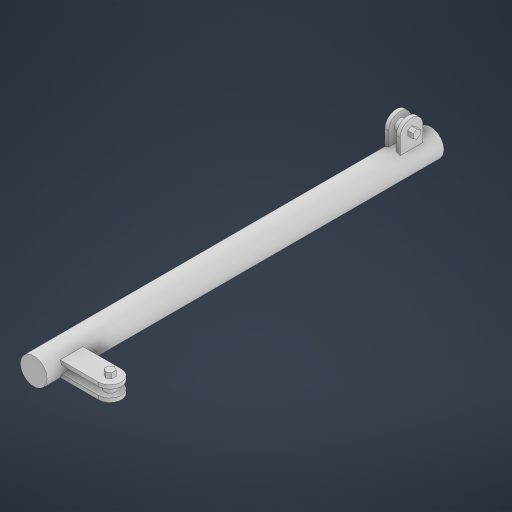
# Autodesk Inventor part: driveshaft_m_mount
Saved by Autodesk Inventor 2023 (Build 270158000, 158)
## iProperties
Created: 2023-09-20
Part Number: driveshaft_m_mount
Material: Generic
Document SubType Name: Modeling
Designer: Peter
Density: 1 g/cm^3
Appearance: Default
Author: Peter
Autodesk Inventor part; units mm, degrees
ref_plane "YZ Plane" through (0, 0, 0) normal (1, 0, 0) x (0, 1, 0)
ref_plane "XZ Plane" through (0, 0, 0) normal (0, 1, 0) x (-1, 0, 0)
ref_plane "XY Plane" through (0, 0, 0) normal (0, 0, 1) x (1, 0, 0)
sketch "Sketch1" plane through (0, 0, 0) normal (0, 0, 1) x (1, 0, 0)
  circle A0 centre (0, 0) radius 44.45
  dimension "d0" = 88.9
  constraints: 1 centre point, 1 coincident
  measures "d0" diameter of A0
extrude "Extrusion1" add sketch "Sketch1" along normal blind 1320.8
sketch "Sketch2" plane through (0, 0, 0) normal (0, 1, 0) x (-1, 0, 0)
  line L0 (12.7, 50.8) -> (25.4, 50.8)
  line L1 (25.4, 50.8) -> (25.4, 127)
  line L2 (25.4, 127) -> (12.7, 127)
  line L3 (12.7, 127) -> (12.7, 50.8)
  line L4 (0, -25.4) -> (0, 152.4) construction
  line L5 (-12.7, 50.8) -> (-25.4, 50.8)
  line L6 (-25.4, 50.8) -> (-25.4, 127)
  line L7 (-25.4, 127) -> (-12.7, 127)
  line L8 (-12.7, 127) -> (-12.7, 50.8)
  point P0 (0, 0)
  dimension "d3" = 76.2
  dimension "d4" = 12.7
  dimension "d5" = 12.7
  dimension "d6" = 50.8
  constraints: 16 end point, 4 symmetric about line, 2 parallel, 1 horizontal, 1 perpendicular
  measures "d3" distance of L0.end L1.end
  measures "d4" distance of L1.end L2.end
  measures "d5" distance between parallel lines of L4 L3
  measures "d6" distance from line of point (0, 0) L0
extrude "Extrusion2" add sketch "Sketch2" along normal blind 127
sketch "Sketch3" plane through (0, 0, 0) normal (1, 0, 0) x (0, 1, 0)
  line L0 (12.7, 1270) -> (25.4, 1270)
  line L1 (25.4, 1270) -> (25.4, 1193.8)
  line L2 (25.4, 1193.8) -> (12.7, 1193.8)
  line L3 (12.7, 1193.8) -> (12.7, 1270)
  line L4 (0, -264.16) -> (0, 1584.96) construction
  line L5 (44.45, 1320.8) -> (-44.45, 1320.8) construction
  line L6 (-12.7, 1270) -> (-25.4, 1270)
  line L7 (-25.4, 1270) -> (-25.4, 1193.8)
  line L8 (-25.4, 1193.8) -> (-12.7, 1193.8)
  line L9 (-12.7, 1193.8) -> (-12.7, 1270)
  point P0 (0, 0)
  point P1 (19.05, 1270)
  point P2 (-19.05, 1270)
  dimension "d10" = 12.7
  dimension "d11" = 12.7
  dimension "d12" = 76.2
  dimension "d13" = 50.8
  constraints: 16 end point, 5 symmetric about line, 2 parallel, 1 horizontal, 1 midpoint, 1 perpendicular
  measures "d10" distance between parallel lines of L4 L3
  measures "d11" distance of L0.start L0.end
  measures "d12" distance of L0.end L1.end
  measures "d13" distance from line of L5 point (19.05, 1270)
extrude "Extrusion3" add sketch "Sketch3" along normal blind 203.2
fillet "Fillet1" radius 38.1 8 edges at (-19.05, 127, 127) (19.05, 127, 127) (19.05, 127, 50.8) (-19.05, 127, 50.8) (203.2, 19.05, 1270) (203.2, 19.05, 1193.8) (203.2, -19.05, 1193.8) (203.2, -19.05, 1270)
sketch "Sketch4" plane through (-12.7, 42.5971, 127) normal (1, 0, 0) x (0, 0, -1)
  arc A0 (76.2, 46.3029) -> (0, 46.3029) centre (38.1, 46.3029) ccw construction
  circle A1 centre (38.1, 46.3029) radius 19.05
  point P0 (127, -42.5971)
  dimension "d16" = 38.1
  constraints: 1 centre point, 1 coincident
  measures "d16" diameter of A1
extrude "Extrusion4" add sketch "Sketch4" along normal up to next
sketch "Sketch5" plane through (42.5971, -12.7, 1270) normal (0, 1, 0) x (1, 0, 0)
  arc A0 (122.5029, 0) -> (122.5029, 76.2) centre (122.5029, 38.1) ccw construction
  circle A1 centre (122.5029, 38.1) radius 19.05
  point P0 (-42.5971, 1270)
  dimension "d19" = 38.1
  constraints: 1 centre point, 1 coincident
  measures "d19" diameter of A1
extrude "Extrusion5" add sketch "Sketch5" along normal blind 25.4
sketch "Sketch6" plane through (25.4, 36.478, 127) normal (1, 0, 0) x (0, 0, -1)
  arc A0 (76.2, 52.422) -> (0, 52.422) centre (38.1, 52.422) ccw construction
  line L0 (38.1, 67.0867) -> (50.8, 59.7544)
  line L1 (50.8, 59.7544) -> (50.8, 45.0897)
  line L2 (50.8, 45.0897) -> (38.1, 37.7573)
  line L3 (38.1, 37.7573) -> (25.4, 45.0897)
  line L4 (25.4, 45.0897) -> (25.4, 59.7544)
  line L5 (25.4, 59.7544) -> (38.1, 67.0867)
  point P0 (127, -36.478)
  point P1 (25.4, 52.422)
  point P2 (50.8, 52.422)
  dimension "d22" = 25.4
  constraints: 12 end point, 2 midpoint, 1 coincident, 13 other
  measures "d22" distance of point (25.4, 52.422) point (50.8, 52.422)
extrude "Extrusion6" add sketch "Sketch6" along normal blind 17.78
sketch "Sketch7" plane through (36.478, 25.4, 1270) normal (0, 1, 0) x (1, 0, 0)
  circle A0 centre (128.622, 38.1) radius 19.05 construction
  line L0 (128.622, 52.7647) -> (141.322, 45.4323)
  line L1 (141.322, 45.4323) -> (141.322, 30.7677)
  line L2 (141.322, 30.7677) -> (128.622, 23.4353)
  line L3 (128.622, 23.4353) -> (115.922, 30.7677)
  line L4 (115.922, 30.7677) -> (115.922, 45.4323)
  line L5 (115.922, 45.4323) -> (128.622, 52.7647)
  point P0 (-36.478, 1270)
  point P1 (115.922, 38.1)
  point P2 (141.322, 38.1)
  dimension "d25" = 25.4
  constraints: 12 end point, 2 midpoint, 1 coincident, 13 other
  measures "d25" distance of point (115.922, 38.1) point (141.322, 38.1)
extrude "Extrusion7" add sketch "Sketch7" along normal blind 17.78
mirror "Mirror2" about plane through (0, 0, 0) normal (0, 1, 0) of "Extrusion7"
mirror "Mirror3" about plane through (0, 0, 0) normal (1, 0, 0) of "Extrusion6"
body "Solid1"
